Autodesk Inventor part; units mm, degrees
(part 2 of 2)
sketch "Эскиз19" plane through (-553.2789, -264.3002, 1.4222) normal (0, -1, 0) x (1, 0, 0)
  line L0 (41.9631, 0) -> (41.9631, -7) projected
  line L1 (41.9631, 0) -> (35.9631, 0) projected
  line L2 (35.9631, -7) -> (35.9631, 0) projected
  line L3 (41.9631, -7) -> (35.9631, -7) projected
  circle A0 centre (38.9631, 8) radius 1.75 projected
  line L4 (41.9631, 23) -> (41.9631, 16) projected
  line L5 (41.9631, 23) -> (35.9631, 23) projected
  line L6 (35.9631, 16) -> (35.9631, 23) projected
  line L7 (41.9631, 16) -> (35.9631, 16) projected
  line L8 (490.3726, 65.8677) -> (-34.6354, 65.8677) projected
  line L9 (35.9631, 109) -> (35.9631, 116) projected
  line L10 (41.9631, 109) -> (35.9631, 109) projected
  line L11 (41.9631, 116) -> (41.9631, 109) projected
  line L12 (35.9631, 116) -> (41.9631, 116) projected
  circle A1 centre (38.9631, 124) radius 1.75 projected
  line L13 (41.9631, 132) -> (35.9631, 132) projected
  line L14 (35.9631, 132) -> (35.9631, 139) projected
  line L15 (35.9631, 139) -> (41.9631, 139) projected
  line L16 (41.9631, 139) -> (41.9631, 132) projected
  line L17 (135.0844, 0) -> (141.0844, 0) projected
  line L18 (135.0844, -7) -> (135.0844, 0) projected
  line L19 (135.3247, -7) -> (136.6297, -7) projected
  line L20 (141.0844, -7) -> (135.0844, -7) projected
  line L21 (141.0844, 0) -> (141.0844, -7) projected
  line L22 (135.0844, 16) -> (135.0844, 23) projected
  line L23 (141.0844, 16) -> (135.0844, 16) projected
  line L24 (141.0844, 23) -> (141.0844, 16) projected
  line L25 (135.0844, 23) -> (141.0844, 23) projected
  circle A2 centre (138.0844, 8) radius 1.75 projected
  line L26 (135.0844, 109) -> (135.0844, 116) projected
  line L27 (135.0844, 116) -> (141.0844, 116) projected
  line L28 (141.0844, 109) -> (135.0844, 109) projected
  line L29 (141.0844, 116) -> (141.0844, 109) projected
  circle A3 centre (138.3833, 122.178) radius 0.9 projected
  circle A4 centre (138.0844, 124) radius 1.75 projected
  line L30 (188.2269, 146.409) -> (188.2269, 95.659) projected
  line L31 (188.2269, 95.659) -> (164.2269, 95.659) projected
  line L32 (164.2269, 95.659) -> (164.2269, 146.409) projected
  line L33 (164.2269, 146.409) -> (188.2269, 146.409) projected
  line L34 (141.0844, 23) -> (141.0844, 16) projected
  line L35 (141.0844, 16) -> (135.0844, 16) projected
  line L36 (135.0844, 16) -> (135.0844, 23) projected
  line L37 (135.0844, 23) -> (141.0844, 23) projected
  line L38 (35.9631, 132) -> (35.9631, 139) projected
  line L39 (35.9631, 139) -> (41.9631, 139) projected
  line L40 (41.9631, 139) -> (41.9631, 132) projected
  line L41 (41.9631, 132) -> (35.9631, 132) projected
  circle A5 centre (38.9631, 8) radius 1.75 projected
  line L42 (41.9631, -7) -> (35.9631, -7) projected
  line L43 (35.9631, -7) -> (35.9631, 0) projected
  line L44 (35.9631, 0) -> (41.9631, 0) projected
  line L45 (41.9631, 0) -> (41.9631, -7) projected
  line L46 (141.0844, 139) -> (141.0844, 132) projected
  line L47 (141.0844, 132) -> (135.0844, 132) projected
  line L48 (135.0844, 132) -> (135.0844, 139) projected
  line L49 (135.0844, 139) -> (141.0844, 139) projected
  circle A6 centre (138.0844, 8) radius 1.75 projected
  line L50 (141.0844, 116) -> (141.0844, 109) projected
  line L51 (141.0844, 109) -> (135.0844, 109) projected
  line L52 (135.0844, 109) -> (135.0844, 116) projected
  line L53 (135.0844, 116) -> (141.0844, 116) projected
  circle A7 centre (38.9631, 124) radius 1.75 projected
  line L54 (41.9631, 16) -> (35.9631, 16) projected
  line L55 (35.9631, 16) -> (35.9631, 23) projected
  line L56 (35.9631, 23) -> (41.9631, 23) projected
  line L57 (41.9631, 23) -> (41.9631, 16) projected
  line L58 (35.9631, 109) -> (35.9631, 116) projected
  line L59 (35.9631, 116) -> (41.9631, 116) projected
  line L60 (41.9631, 116) -> (41.9631, 109) projected
  line L61 (41.9631, 109) -> (35.9631, 109) projected
  circle A8 centre (138.0844, 124) radius 1.75 projected
  line L62 (141.0844, 0) -> (141.0844, -7) projected
  line L63 (141.0844, -7) -> (135.0844, -7) projected
  line L64 (135.0844, -7) -> (135.0844, 0) projected
  line L65 (135.0844, 0) -> (141.0844, 0) projected
  circle A9 centre (130.9111, -16.5023) radius 1.2859 projected
  circle A10 centre (209.5461, 19.0176) radius 1.3005 projected
  circle A11 centre (130.9552, 19.0345) radius 1.2516 projected
  circle A12 centre (209.4904, -16.5085) radius 1.3414 projected
  circle A13 centre (194.5237, 85.5) radius 1.6 projected
  spline S0 degree 3 poles (38.7737, 66.1) (38.7737, 66.2887) (38.8115, 66.4898) (38.9647, 66.8592) (39.0801, 67.0277) (39.3461, 67.2936) (39.5145, 67.409) (39.884, 67.5622) (40.085, 67.6) (40.4625, 67.6) (40.6635, 67.5622) (41.033, 67.409) (41.2014, 67.2936) (41.4674, 67.0277) (41.5828, 66.8592) (41.7359, 66.4898) (41.7737, 66.2887) (41.7737, 65.9113) (41.7359, 65.7102) (41.5828, 65.3408) (41.4674, 65.1723) (41.2014, 64.9064) (41.033, 64.791) (40.6635, 64.6378) (40.4625, 64.6) (40.085, 64.6) (39.884, 64.6378) (39.5145, 64.791) (39.3461, 64.9064) (39.0801, 65.1723) (38.9647, 65.3408) (38.8115, 65.7102) (38.7737, 65.9113) (38.7737, 66.1) knots 0 0 0 0 0.056617 0.056617 0.113235 0.113235 0.169851 0.169851 0.226467 0.226467 0.283083 0.283083 0.339699 0.339699 0.396316 0.396316 0.452934 0.452934 0.509551 0.509551 0.566168 0.566168 0.622784 0.622784 0.6794 0.6794 0.736016 0.736016 0.792632 0.792632 0.84925 0.84925 0.905867 0.905867 0.905867 0.905867 projected
  spline S1 degree 3 poles (-19.7263, 65.9) (-19.7263, 65.7113) (-19.7641, 65.5102) (-19.9172, 65.1408) (-20.0326, 64.9723) (-20.2986, 64.7064) (-20.467, 64.591) (-20.8365, 64.4378) (-21.0375, 64.4) (-21.415, 64.4) (-21.616, 64.4378) (-21.9855, 64.591) (-22.1539, 64.7064) (-22.4199, 64.9723) (-22.5353, 65.1408) (-22.6885, 65.5102) (-22.7263, 65.7113) (-22.7263, 66.0887) (-22.6885, 66.2898) (-22.5353, 66.6592) (-22.4199, 66.8277) (-22.1539, 67.0936) (-21.9855, 67.209) (-21.616, 67.3622) (-21.415, 67.4) (-21.0375, 67.4) (-20.8365, 67.3622) (-20.467, 67.209) (-20.2986, 67.0936) (-20.0326, 66.8277) (-19.9172, 66.6592) (-19.7641, 66.2898) (-19.7263, 66.0887) (-19.7263, 65.9) knots 0 0 0 0 0.056617 0.056617 0.113235 0.113235 0.169851 0.169851 0.226467 0.226467 0.283083 0.283083 0.339699 0.339699 0.396316 0.396316 0.452934 0.452934 0.509551 0.509551 0.566168 0.566168 0.622784 0.622784 0.6794 0.6794 0.736016 0.736016 0.792632 0.792632 0.84925 0.84925 0.905867 0.905867 0.905867 0.905867 projected
  circle A14 centre (132.5237, 149.5) radius 1.6 projected
  circle A15 centre (132.5237, 37.5) radius 1.6 projected
  circle A16 centre (132.5237, 85.5) radius 1.6 projected
  spline S2 degree 3 poles (21.2737, 65.9) (21.2737, 65.7113) (21.2359, 65.5102) (21.0828, 65.1408) (20.9674, 64.9723) (20.7014, 64.7064) (20.533, 64.591) (20.1635, 64.4378) (19.9625, 64.4) (19.585, 64.4) (19.384, 64.4378) (19.0145, 64.591) (18.8461, 64.7064) (18.5801, 64.9723) (18.4647, 65.1408) (18.3115, 65.5102) (18.2737, 65.7113) (18.2737, 66.0887) (18.3115, 66.2898) (18.4647, 66.6592) (18.5801, 66.8277) (18.8461, 67.0936) (19.0145, 67.209) (19.384, 67.3622) (19.585, 67.4) (19.9625, 67.4) (20.1635, 67.3622) (20.533, 67.209) (20.7014, 67.0936) (20.9674, 66.8277) (21.0828, 66.6592) (21.2359, 66.2898) (21.2737, 66.0887) (21.2737, 65.9) knots 0 0 0 0 0.056617 0.056617 0.113235 0.113235 0.169851 0.169851 0.226467 0.226467 0.283083 0.283083 0.339699 0.339699 0.396316 0.396316 0.452934 0.452934 0.509551 0.509551 0.566168 0.566168 0.622784 0.622784 0.6794 0.6794 0.736016 0.736016 0.792632 0.792632 0.84925 0.84925 0.905867 0.905867 0.905867 0.905867 projected
  spline S3 degree 3 poles (-2.2263, 66.1) (-2.2263, 66.2887) (-2.1885, 66.4898) (-2.0353, 66.8592) (-1.9199, 67.0277) (-1.6539, 67.2936) (-1.4855, 67.409) (-1.116, 67.5622) (-0.915, 67.6) (-0.5375, 67.6) (-0.3365, 67.5622) (0.033, 67.409) (0.2014, 67.2936) (0.4674, 67.0277) (0.5828, 66.8592) (0.7359, 66.4898) (0.7737, 66.2887) (0.7737, 65.9113) (0.7359, 65.7102) (0.5828, 65.3408) (0.4674, 65.1723) (0.2014, 64.9064) (0.033, 64.791) (-0.3365, 64.6378) (-0.5375, 64.6) (-0.915, 64.6) (-1.116, 64.6378) (-1.4855, 64.791) (-1.6539, 64.9064) (-1.9199, 65.1723) (-2.0353, 65.3408) (-2.1885, 65.7102) (-2.2263, 65.9113) (-2.2263, 66.1) knots 0 0 0 0 0.056617 0.056617 0.113235 0.113235 0.169851 0.169851 0.226467 0.226467 0.283083 0.283083 0.339699 0.339699 0.396316 0.396316 0.452934 0.452934 0.509551 0.509551 0.566168 0.566168 0.622784 0.622784 0.6794 0.6794 0.736016 0.736016 0.792632 0.792632 0.84925 0.84925 0.905867 0.905867 0.905867 0.905867 projected
  circle A17 centre (194.5237, 149.5) radius 1.6 projected
  circle A18 centre (194.5237, 37.5) radius 1.6 projected
  line L66 (18.5237, 115.5) -> (18.5237, 105.5) projected
  line L67 (18.5237, 105.5) -> (-26.4763, 105.5) projected
  line L68 (-26.4763, 105.5) -> (-26.4763, 115.5) projected
  line L69 (-26.4763, 115.5) -> (18.5237, 115.5) projected
  line L70 (18.5237, 26.5) -> (18.5237, 16.5) projected
  line L71 (18.5237, 16.5) -> (-26.4763, 16.5) projected
  line L72 (-26.4763, 16.5) -> (-26.4763, 26.5) projected
  line L73 (-26.4763, 26.5) -> (18.5237, 26.5) projected
  circle A19 centre (0, -28.25) radius 1.75 projected
  circle A20 centre (0, 160.25) radius 1.75 projected
  circle A21 centre (195.0475, 160.25) radius 1.75 projected
  circle A22 centre (195.0475, -28.25) radius 1.75 projected
  circle A23 centre (177.0475, 160.25) radius 1.75 projected
  circle A24 centre (-18, 160.25) radius 1.75 projected
  circle A25 centre (-18, -28.25) radius 1.75 projected
  circle A26 centre (18, 160.25) radius 1.75 projected
  circle A27 centre (159.0475, -28.25) radius 1.75 projected
  circle A28 centre (177.0475, -28.25) radius 1.75 projected
  circle A29 centre (159.0475, 160.25) radius 1.75 projected
  circle A30 centre (18, -28.25) radius 1.75 projected
  circle A31 centre (53.5237, 156) radius 5 projected
  circle A32 centre (53.5237, -24) radius 5 projected
  line L74 (66.0237, 157.5) -> (111.0237, 157.5) projected
  line L75 (111.0237, 157.5) -> (111.0237, -25.5) projected
  line L76 (111.0237, -25.5) -> (66.0237, -25.5) projected
  line L77 (66.0237, -25.5) -> (66.0237, 157.5) projected
  line L78 (204.5237, 93.5765) -> (216.5237, 93.5765) projected
  line L79 (216.5237, 93.5765) -> (216.5237, 38.5765) projected
  line L80 (216.5237, 38.5765) -> (204.5237, 38.5765) projected
  line L81 (204.5237, 38.5765) -> (204.5237, 93.5765) projected
  circle A33 centre (-43.4763, 18.5) radius 1.75 projected
  circle A34 centre (-43.4763, 55.625) radius 1.75 projected
  circle A35 centre (-43.4763, 113.5) radius 1.75 projected
  circle A36 centre (-43.4763, 76.375) radius 1.75 projected
  arc A37 (-38.4763, 163.5) -> (-46.4763, 155.5) centre (-38.4763, 155.5) ccw projected
  line L82 (-46.4763, 155.5) -> (-46.4763, 143.5) projected
  line L83 (-46.4763, 143.5) -> (-40.4763, 143.5) projected
  line L84 (-40.4763, 143.5) -> (-40.4763, 123.5) projected
  line L85 (-40.4763, 123.5) -> (-46.4763, 123.5) projected
  line L86 (-46.4763, 123.5) -> (-46.4763, 103.5) projected
  line L87 (-46.4763, 103.5) -> (-40.4763, 103.5) projected
  line L88 (-40.4763, 103.5) -> (-40.4763, 83.5) projected
  line L89 (-40.4763, 83.5) -> (-46.4763, 83.5) projected
  line L90 (-46.4763, 83.5) -> (-46.4763, 48.5) projected
  line L91 (-46.4763, 48.5) -> (-40.4763, 48.5) projected
  line L92 (-40.4763, 48.5) -> (-40.4763, 28.5) projected
  line L93 (-40.4763, 28.5) -> (-46.4763, 28.5) projected
  line L94 (-46.4763, 28.5) -> (-46.4763, 8.5) projected
  line L95 (-46.4763, 8.5) -> (-40.4763, 8.5) projected
  line L96 (-40.4763, 8.5) -> (-40.4763, -11.5) projected
  line L97 (-40.4763, -11.5) -> (-46.4763, -11.5) projected
  line L98 (-46.4763, -11.5) -> (-46.4763, -23.5) projected
  arc A38 (-46.4763, -23.5) -> (-38.4763, -31.5) centre (-38.4763, -23.5) ccw projected
  line L99 (-38.4763, -31.5) -> (26, -31.5) projected
  arc A39 (30, -35.5) -> (26, -31.5) centre (22.7085, -38.7915) ccw projected
  line L100 (30, -35.5) -> (30, -39) projected
  arc A40 (30, -39) -> (38, -47) centre (38, -39) ccw projected
  line L101 (38, -47) -> (138.803, -47) projected
  arc A41 (138.803, -47) -> (146.803, -39) centre (138.803, -39) ccw projected
  line L102 (146.803, -39) -> (146.803, -35.5) projected
  arc A42 (150.803, -31.5) -> (146.803, -35.5) centre (154.0945, -38.7915) ccw projected
  line L103 (150.803, -31.5) -> (215.5237, -31.5) projected
  arc A43 (215.5237, -31.5) -> (223.5237, -23.5) centre (215.5237, -23.5) ccw projected
  line L104 (223.5237, -23.5) -> (223.5237, 155.5) projected
  arc A44 (223.5237, 155.5) -> (215.5237, 163.5) centre (215.5237, 155.5) ccw projected
  line L105 (215.5237, 163.5) -> (150.803, 163.5) projected
  arc A45 (146.803, 167.7701) -> (150.803, 163.5) centre (154.2371, 170.7254) ccw projected
  line L106 (146.803, 167.7701) -> (146.803, 171.2701) projected
  arc A46 (146.803, 171.2701) -> (138.803, 179.2701) centre (138.803, 171.2701) ccw projected
  line L107 (138.803, 179.2701) -> (38.2701, 179.2701) projected
  arc A47 (38.2701, 179.2701) -> (30.2701, 171.2701) centre (38.2701, 171.2701) ccw projected
  line L108 (30.2701, 171.2701) -> (30.2701, 167.7701) projected
  arc A48 (26, 163.5) -> (30.2701, 167.7701) centre (22.8966, 170.8735) ccw projected
  line L109 (26, 163.5) -> (-38.4763, 163.5) projected
  circle A49 centre (111.0237, -35.5) radius 2 projected
  circle A50 centre (88.5237, -35.5) radius 2 projected
  circle A51 centre (66.0237, -35.5) radius 2 projected
  circle A52 centre (111.0237, 167.5) radius 2 projected
  circle A53 centre (88.5237, 167.5) radius 2 projected
  circle A54 centre (66.0237, 167.5) radius 2 projected
  point P0 (553.2789, -1.4222)
  point P1 (135.3367, -1.987)
  point P2 (38.7737, 66.1)
  point P3 (-19.7263, 65.9)
  point P4 (21.2737, 65.9)
  point P5 (-2.2263, 66.1)
  constraints: 2 other
extrude "Выдавливание18" cut sketch "Эскиз19" against normal blind 8 contours L0 L3 L2 L1 | A0 | L4 L7 L6 L5 | L9 L12 L11 L10 | A1 | L13 L14 L15 L16 | L17 L21 L20 L19 L18 | L22 L25 L24 L23 | A2 | L26 L27 L29 L28 | A4 A3 | A3 A4 | L46 L47 L48 L49 picked at (138.3234, 122.5433) picked at (137.848, 124.8105)
sketch "Эскиз20" plane through (-553.2789, -264.3002, 1.4222) normal (0, -1, 0) x (1, 0, 0)
  spline S0 degree 3 poles (186.0428, -20.0009) (186.0418, -20.0863) (186.047, -20.2644) (186.1773, -20.7176) (186.2643, -20.9293) (186.5878, -21.4217) (186.8123, -21.5786) (187.0607, -21.7563) (187.2804, -21.8685) (187.7436, -21.9734) (188.0102, -22.0137) (188.2767, -21.9939) (188.596, -21.9503) (189.2286, -21.6371) (189.3773, -21.5085) (189.6736, -21.2131) (189.7882, -21.0138) (189.9687, -20.5892) (190.0251, -20.3525) (190.0563, -20.0478) (190.0583, -19.763) (189.8274, -19.0006) (189.666, -18.8178) (189.5078, -18.6264) (189.3722, -18.4844) (188.8741, -18.1265) (188.4982, -18.0562) (188.1379, -17.9726) (187.9735, -17.9836) (187.5992, -18.0475) (187.3221, -18.1305) (186.9314, -18.3252) (186.7276, -18.4693) (186.3253, -18.9343) (186.2291, -19.139) (186.1035, -19.5227) (186.0453, -19.7803) (186.0428, -20.0009) knots -0.617581 -0.617581 -0.617581 -0.617581 -0.591947 -0.591947 -0.573073 -0.573073 -0.540222 -0.540222 -0.491682 -0.491682 -0.466072 -0.466072 -0.460987 -0.460987 -0.456841 -0.456841 -0.449459 -0.449459 -0.440712 -0.440712 -0.435051 -0.435051 -0.427631 -0.427631 -0.418066 -0.418066 -0.393854 -0.393854 -0.318016 -0.318016 -0.225773 -0.225773 -0.149383 -0.149383 -0.066183 -0.066183 0 0 0 0 projected
  spline S1 degree 3 poles (164.0117, -21.2982) (164.169, -21.4756) (164.4102, -21.6815) (164.8908, -21.917) (165.1232, -21.9678) (165.5486, -22.0096) (165.8027, -22.0092) (166.4276, -21.8156) (166.6468, -21.6708) (167.1153, -21.2784) (167.2685, -20.9945) (167.3708, -20.7958) (167.4641, -20.5667) (167.5376, -20.1343) (167.5565, -19.8881) (167.4331, -19.3599) (167.3466, -19.0991) (167.0265, -18.6518) (166.8426, -18.4698) (166.358, -18.1486) (166.0886, -18.0712) (165.5758, -17.973) (165.3134, -18.003) (164.9711, -18.0757) (164.755, -18.1419) (164.4662, -18.2967) (164.2497, -18.4223) (163.8791, -18.878) (163.7442, -19.0633) (163.6277, -19.3522) (163.5369, -19.5835) (163.5364, -20.3503) (163.6125, -20.5971) (163.8043, -21.0552) (163.9656, -21.2462) (164.0117, -21.2982) knots -1.840358 -1.840358 -1.840358 -1.840358 -1.769222 -1.769222 -1.709875 -1.709875 -1.656566 -1.656566 -1.604902 -1.604902 -1.500987 -1.500987 -1.176684 -1.176684 -0.960047 -0.960047 -0.825926 -0.825926 -0.728108 -0.728108 -0.603604 -0.603604 -0.389887 -0.389887 -0.189621 -0.189621 -0.087541 -0.087541 -0.045854 -0.045854 -0.032602 -0.032602 -0.020855 -0.020855 0 0 0 0 projected
  spline S2 degree 3 poles (186.0428, 152.0009) (186.0418, 152.0863) (186.047, 152.2644) (186.1773, 152.7176) (186.2643, 152.9293) (186.5878, 153.4217) (186.8123, 153.5786) (187.0607, 153.7563) (187.2804, 153.8685) (187.7436, 153.9734) (188.0102, 154.0137) (188.2767, 153.9939) (188.596, 153.9503) (189.2286, 153.6371) (189.3773, 153.5085) (189.6736, 153.2131) (189.7882, 153.0138) (189.9687, 152.5892) (190.0251, 152.3525) (190.0563, 152.0478) (190.0583, 151.763) (189.8274, 151.0006) (189.666, 150.8178) (189.5078, 150.6264) (189.3722, 150.4844) (188.8741, 150.1265) (188.4982, 150.0562) (188.1379, 149.9726) (187.9735, 149.9837) (187.5992, 150.0475) (187.3221, 150.1305) (186.9314, 150.3252) (186.7276, 150.4693) (186.3253, 150.9343) (186.2291, 151.139) (186.1035, 151.5227) (186.0453, 151.7803) (186.0428, 152.0009) knots -0.617581 -0.617581 -0.617581 -0.617581 -0.591947 -0.591947 -0.573073 -0.573073 -0.540222 -0.540222 -0.491682 -0.491682 -0.466072 -0.466072 -0.460987 -0.460987 -0.456841 -0.456841 -0.449459 -0.449459 -0.440712 -0.440712 -0.435051 -0.435051 -0.427631 -0.427631 -0.418066 -0.418066 -0.393854 -0.393854 -0.318016 -0.318016 -0.225773 -0.225773 -0.149383 -0.149383 -0.066183 -0.066183 0 0 0 0 projected
  spline S3 degree 3 poles (164.0117, 153.2982) (164.169, 153.4756) (164.4102, 153.6815) (164.8908, 153.917) (165.1232, 153.9678) (165.5486, 154.0096) (165.8027, 154.0092) (166.4276, 153.8156) (166.6468, 153.6708) (167.1153, 153.2785) (167.2685, 152.9945) (167.3708, 152.7958) (167.4641, 152.5667) (167.5376, 152.1343) (167.5565, 151.8881) (167.4331, 151.3599) (167.3466, 151.0991) (167.0265, 150.6518) (166.8426, 150.4698) (166.358, 150.1486) (166.0886, 150.0712) (165.5758, 149.973) (165.3134, 150.003) (164.9711, 150.0757) (164.755, 150.1419) (164.4662, 150.2968) (164.2497, 150.4223) (163.8791, 150.878) (163.7442, 151.0633) (163.6277, 151.3522) (163.5369, 151.5835) (163.5364, 152.3503) (163.6125, 152.5972) (163.8043, 153.0552) (163.9656, 153.2462) (164.0117, 153.2982) knots -1.840358 -1.840358 -1.840358 -1.840358 -1.769222 -1.769222 -1.709875 -1.709875 -1.656566 -1.656566 -1.604902 -1.604902 -1.500987 -1.500987 -1.176684 -1.176684 -0.960047 -0.960047 -0.825926 -0.825926 -0.728108 -0.728108 -0.603604 -0.603604 -0.389887 -0.389887 -0.189621 -0.189621 -0.087541 -0.087541 -0.045854 -0.045854 -0.032602 -0.032602 -0.020855 -0.020855 0 0 0 0 projected
  point P0 (553.2789, -1.4222)
  point P1 (186.0428, -20.0009)
  point P2 (164.0117, -21.2982)
  point P3 (186.0428, 152.0009)
  point P4 (164.0117, 153.2982)
extrude "Выдавливание19" cut sketch "Эскиз20" against normal blind 10
sketch "Эскиз21" plane through (-553.2789, -260.3002, 1.4222) normal (0, 1, 0) x (1, 0, 0)
  circle A0 centre (20.333, -160.5) radius 2 projected
  circle A1 centre (20.333, -140.5) radius 2 projected
  circle A2 centre (-3.667, -160.5) radius 2 projected
  circle A3 centre (-3.667, -140.5) radius 2 projected
  circle A4 centre (20.333, 8.5) radius 2 projected
  circle A5 centre (20.333, 28.5) radius 2 projected
  circle A6 centre (-3.667, 8.5) radius 2 projected
  circle A7 centre (-3.667, 28.5) radius 2 projected
  point P0 (553.2789, 1.4222)
extrude "Выдавливание20" cut sketch "Эскиз21" against normal blind 10
